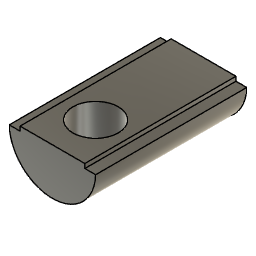
PTC-HRNM5 v1 (Autodesk Fusion 360 design; units mm, degrees)
Autodesk Fusion 360 part; units mm, degrees
sketch "Sketch1" plane through (0, 0, 0) normal (0, 1, 0) x (1, 0, 0)
  line L0 (0, 0) -> (0, -4.3) construction
  line L1 (3, -4.3) -> (-3, -4.3)
  line L2 (3, -4.3) -> (3, -3.9)
  line L3 (3, -3.9) -> (4, -3.9)
  line L4 (-3, -4.3) -> (-3, -3.9)
  line L5 (-3, -3.9) -> (-4, -3.9)
  circle A0 centre (0, -4.0013) radius 4.0013
  dimension "d1" = 4.3
  dimension "d3" = 6
  dimension "d4" = 0.4
  dimension "d5" = 1
  dimension "d6" = 0.4
  dimension "d7" = 1
  constraint coincident L0.start origin
  constraint vertical L0
  constraint perpendicular L0 L1
  constraint perpendicular L1 L2
  constraint perpendicular L2 L3
  constraint perpendicular L1 L4
  constraint perpendicular L4 L5
  constraint coincident L0.start A0
  constraint coincident L3.end A0
  constraint coincident L5.end A0
  measures "d1" distance of L0.start L0.end
  measures "d3" distance of L1.start L1.end
  measures "d4" distance of L1.start L2.end
  measures "d5" distance of L2.end L3.end
  measures "d6" distance of L1.end L4.end
  measures "d7" distance of L4.end L5.end
extrude "Extrude1" add sketch "Sketch1" along normal mid plane 14 contours L1 L2 L3 L4 L5 A0 picked at (0.0981, -2.6036)
sketch "Sketch2" plane through (0, 0, 4.3) normal (0, 0, 1) x (-1, 0, 0)
  line L0 (-3, 7) -> (-3, -7)
  line L1 (-3, -7) -> (3, -7)
  line L2 (3, -7) -> (3, 7)
  line L3 (3, 7) -> (-3, 7)
  line L4 (0, 7) -> (0, 3) construction
  dimension "d10" = 4
  constraint midpoint L3 L4.start
  constraint perpendicular L3 L4
  measures "d10" distance of L4.start L4.end
hole "Hole1" at (0, -3, 4.3) direction (0, 0, -1) diameter 4.2 depth 4.3 tip angle 180
